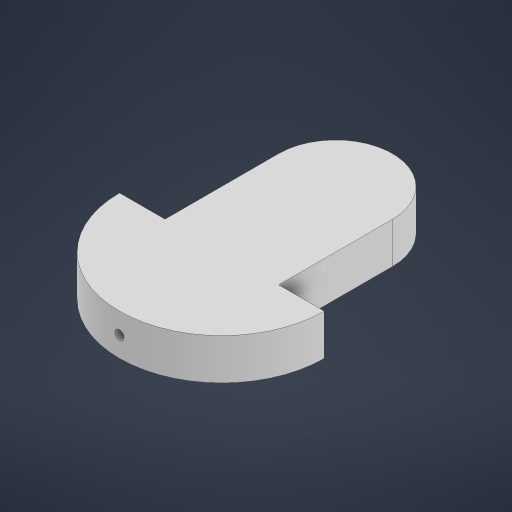
# Autodesk Inventor part: APM_001-1
Saved by Autodesk Inventor 2024 (Build 280153000, 153)
## iProperties
Created: 2023-05-12
Part Number: APM_001-1
Material: Genérico
Document SubType Name: Modeling
Designer: javie
Density: 1 g/cm^3
Appearance: Valor por defecto
Author: javie
Autodesk Inventor part; units mm, degrees
ref_plane "YZ Plane" through (0, 0, 0) normal (1, 0, 0) x (0, 1, 0)
ref_plane "XZ Plane" through (0, 0, 0) normal (0, 1, 0) x (-1, 0, 0)
ref_plane "XY Plane" through (0, 0, 0) normal (0, 0, 1) x (1, 0, 0)
sketch "Boceto1" plane through (0, 0, 0) normal (0, 1, 0) x (-1, 0, 0)
  arc A0 (-25, 25) -> (25, 25) centre (0, 25) ccw
  arc A1 (45, 75) -> (-45, 75) centre (0, 75) ccw
  line L0 (25, 25) -> (25, 75)
  line L1 (-25, 25) -> (-25, 75)
  line L2 (45, 75) -> (25, 75)
  line L3 (-25, 75) -> (-45, 75)
  point P0 (0, 0)
  dimension "d3" = 50
  dimension "d4" = 90
  constraints: 8 end point, 4 point on circle, 2 centre point, 2 perpendicular, 1 parallel
  measures "d3" diameter of A0
  measures "d4" diameter of A1
extrude "Extrusión1" add sketch "Boceto1" along normal blind 18
ref_plane "Plano de trabajo2" through (0, 0, 120) normal (0, 0, -1) x (-1, 0, 0)
sketch "Boceto2" plane through (0, 0, 120) normal (0, 0, -1) x (-1, 0, 0)
  circle A0 centre (0, 9) radius 2
  line L0 (45, 0) -> (-45, 0) projected
  point P0 (0, 0)
  dimension "d9" = 4
  dimension "d10" = 9
  constraints: 1 centre point
  measures "d9" diameter of A0
  measures "d10" distance from line of L0 A0.centre
extrude "Extrusión2" cut sketch "Boceto2" along normal through all
